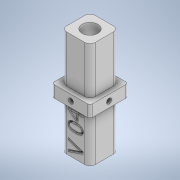
# Autodesk Inventor part: Supports
Saved by Autodesk Inventor 2020 (Build 240168000, 168)
## iProperties
Created: 2019-07-12
Part Number: Supports
Material: Generic
Document SubType Name: Modeling
Designer: steele
Density: 1 g/cm^3
Appearance: Default
Author: steele
Autodesk Inventor part; units mm, degrees
ref_plane "YZ Plane" through (0, 0, 0) normal (1, 0, 0) x (0, 1, 0)
ref_plane "XZ Plane" through (0, 0, 0) normal (0, 1, 0) x (-1, 0, 0)
ref_plane "XY Plane" through (0, 0, 0) normal (0, 0, 1) x (1, 0, 0)
sketch "Sketch1" plane through (0, 0, 0) normal (0, 1, 0) x (-1, 0, 0)
  line L0 (11.43, 11.43) -> (-11.43, 11.43)
  line L1 (-11.43, 11.43) -> (-11.43, -11.43)
  line L2 (-11.43, -11.43) -> (11.43, -11.43)
  line L3 (11.43, -11.43) -> (11.43, 11.43)
  line L4 (11.43, 11.43) -> (-11.43, -11.43) construction
  line L5 (-11.43, 11.43) -> (11.43, -11.43) construction
  point P0 (0, 0)
  dimension "outerWidth" = 22.86
  dimension "outerLength" = 22.86
  constraints: 12 end point, 2 midpoint, 2 parallel, 1 horizontal, 1 perpendicular
  measures "outerWidth" distance of L0.start L0.end
  measures "outerLength" distance of L1.end L0.end
extrude "Extrusion1" add sketch "Sketch1" along normal mid plane 7.112
sketch "Sketch2" plane through (0, 0, 0) normal (0, 1, 0) x (-1, 0, 0)
  line L0 (8.5725, 8.5725) -> (-8.5725, 8.5725)
  line L1 (-8.5725, 8.5725) -> (-8.5725, -8.5725)
  line L2 (-8.5725, -8.5725) -> (8.5725, -8.5725)
  line L3 (8.5725, -8.5725) -> (8.5725, 8.5725)
  line L4 (8.5725, 8.5725) -> (-8.5725, -8.5725) construction
  line L5 (-8.5725, 8.5725) -> (8.5725, -8.5725) construction
  point P0 (0, 0)
  dimension "innerWidth" = 17.145
  dimension "innerLength" = 17.145
  constraints: 12 end point, 2 midpoint, 2 parallel, 1 horizontal, 1 perpendicular
  measures "innerWidth" distance of L0.start L0.end
  measures "innerLength" distance of L1.end L0.end
extrude "Extrusion2" add sketch "Sketch2" along normal mid plane 63.5
sketch "Sketch3" plane through (-8.5725, -3.556, 8.5725) normal (0, 0, 1) x (1, 0, 0)
  line L0 (0, -28.194) -> (17.145, -28.194) construction
  line L1 (13.0175, -28.194) -> (13.0175, 0) construction
  line L2 (20.0025, 0) -> (-2.8575, 0) construction
  line L3 (17.145, 0) -> (17.145, -28.194) projected
  line L4 (4.1275, -18.9779) -> (13.0175, -22.0396)
  line L5 (13.0175, -22.0396) -> (13.0175, -23.3148)
  line L6 (13.0175, -23.3148) -> (4.1275, -26.3766)
  line L7 (4.1275, -26.3766) -> (4.1275, -25.1086)
  line L8 (4.1275, -25.1086) -> (11.5118, -22.6448)
  line L9 (11.5118, -22.6448) -> (4.1275, -20.181)
  line L10 (4.1275, -20.181) -> (4.1275, -18.9779)
  spline S0 degree 2 poles (8.5725, -8.928) (10.9643, -8.928) (13.2048, -10.3184) (13.2048, -11.7664) knots 0 0 0 1 2 2 2
  spline S1 degree 2 poles (13.2048, -11.7664) (13.2048, -13.2361) (10.9211, -14.6121) (8.5797, -14.6121) knots 0 0 0 1 2 2 2
  spline S2 degree 2 poles (8.5797, -14.6121) (6.1735, -14.6121) (3.9474, -13.2217) (3.9474, -11.7664) knots 0 0 0 1 2 2 2
  spline S3 degree 2 poles (3.9474, -11.7664) (3.9474, -10.304) (6.2527, -8.928) (8.5725, -8.928) knots 0 0 0 1 2 2 2
  spline S4 degree 2 poles (11.2813, -10.4553) (10.8418, -10.2824) (9.4874, -10.1383) (8.5725, -10.1383) knots 0 0 0 1 2 2 2
  spline S5 degree 2 poles (8.5725, -10.1383) (7.6576, -10.1383) (6.3104, -10.2824) (5.8565, -10.4625) knots 0 0 0 1 2 2 2
  spline S6 degree 2 poles (5.8565, -10.4625) (5.4026, -10.6426) (4.9344, -11.2693) (4.9344, -11.7664) knots 0 0 0 1 2 2 2
  spline S7 degree 2 poles (4.9344, -11.7664) (4.9344, -12.2635) (5.4026, -12.9047) (5.8709, -13.092) knots 0 0 0 1 2 2 2
  spline S8 degree 2 poles (5.8709, -13.092) (6.3248, -13.2721) (7.708, -13.4018) (8.5797, -13.4018) knots 0 0 0 1 2 2 2
  spline S9 degree 2 poles (8.5797, -13.4018) (9.5163, -13.4018) (10.7698, -13.2865) (11.2597, -13.0992) knots 0 0 0 1 2 2 2
  spline S10 degree 2 poles (11.2597, -13.0992) (11.7207, -12.9263) (12.2178, -12.2851) (12.2178, -11.7664) knots 0 0 0 1 2 2 2
  spline S11 degree 2 poles (12.2178, -11.7664) (12.2178, -11.2766) (11.7496, -10.6354) (11.2813, -10.4553) knots 0 0 0 1 2 2 2
  line L11 (9.9629, -2.0696) -> (9.9629, -3.1286)
  line L12 (9.9629, -3.1286) -> (13.0175, -3.1286)
  line L13 (13.0175, -3.1286) -> (13.0175, -4.2741)
  line L14 (13.0175, -4.2741) -> (9.9629, -4.2741)
  line L15 (9.9629, -4.2741) -> (9.9629, -8.2004)
  line L16 (9.9629, -8.2004) -> (8.7094, -8.2004)
  line L17 (8.7094, -8.2004) -> (4.1275, -4.2236)
  line L18 (4.1275, -4.2236) -> (4.1275, -3.1286)
  line L19 (4.1275, -3.1286) -> (9.0048, -3.1286)
  line L20 (9.0048, -3.1286) -> (9.0048, -2.0696)
  line L21 (9.0048, -2.0696) -> (9.9629, -2.0696)
  line L22 (9.0048, -4.2741) -> (5.5323, -4.2741)
  line L23 (5.5323, -4.2741) -> (9.0048, -7.2638)
  line L24 (9.0048, -7.2638) -> (9.0048, -4.2741)
  point P0 (8.5725, 3.556)
  dimension "textCenterLine" = 4.1275
  constraints: 2 end point, 2 point on line, 2 vertical
  measures "textCenterLine" distance between parallel lines of L3 L1
extrude "Extrusion4" cut sketch "Sketch3" against normal blind 2.54
sketch "Sketch4" plane through (0, 31.75, 0) normal (0, 1, 0) x (1, 0, 0)
  point P0 (0, 0)
  point P1 (0, 0)
  constraints: 1 coincident
hole "Hole1" at (0, 31.75, 0) direction (0, -1, 0) diameter 9.525 end through all
fillet "Fillet1" radius 1.5875 4 edges at (-11.43, 0, 11.43) (11.43, 0, 11.43) (11.43, 0, -11.43) (-11.43, 0, -11.43)
fillet "Fillet2" radius 3.175 8 edges at (8.5725, 17.653, -8.5725) (8.5725, 17.653, 8.5725) (-8.5725, 17.653, -8.5725) (-8.5725, 17.653, 8.5725) (8.5725, -17.653, -8.5725) (8.5725, -17.653, 8.5725) (-8.5725, -17.653, -8.5725) (-8.5725, -17.653, 8.5725)
sketch "Sketch5" plane through (-9.8425, 3.556, 11.43) normal (0, 0, 1) x (1, 0, 0)
  point P0 (9.8425, -3.556)
  point P1 (9.8425, -3.556)
  constraints: 1 coincident
sketch "Sketch6" plane through (11.43, -3.556, -9.8425) normal (1, 0, 0) x (0, 0, -1)
  point P0 (-9.8425, 3.556)
  point P1 (-9.8425, 3.556)
  constraints: 1 coincident
sketch "Sketch7" plane through (9.8425, 3.556, -11.43) normal (0, 0, -1) x (-1, 0, 0)
  point P0 (9.8425, -3.556)
  point P1 (9.8425, -3.556)
  constraints: 1 coincident
sketch "Sketch8" plane through (-11.43, -3.556, -9.8425) normal (-1, 0, 0) x (0, 0, 1)
  point P0 (9.8425, 3.556)
  point P1 (9.8425, 3.556)
  constraints: 1 coincident
hole "Hole2" at (0, 0, 11.43) direction (0, 0, -1) diameter 3.048 depth 12.7 tip angle 118
hole "Hole3" at (11.43, 0, 0) direction (-1, 0, 0) diameter 3.048 depth 12.7 tip angle 118
hole "Hole4" at (0, 0, -11.43) direction (0, 0, 1) diameter 3.048 depth 12.7 tip angle 118
hole "Hole5" at (-11.43, 0, 0) direction (1, 0, 0) diameter 3.048 depth 12.7 tip angle 118
equation "\"textCenterLine\" = 0.5 * innerWidth - 0.5 * textHeight"
equation "\"textHeight\" = 8.89"
body "Solid1"
